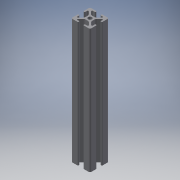
# Autodesk Inventor part: 25-2525_165mm
Saved by Autodesk Inventor 2019.4 (Build 234330000, 330)
## iProperties
Company: 80/20 Inc.
Created: 2014-04-23
Part Number: 25-2525_165mm
Material: Generic
Document SubType Name: Modeling
Designer: Ross Bowman
Density: 1 g/cm^3
Engineer: Ross Bowman
Catalog Web Link: 8020.net
Vendor: 80/20 Inc.
Appearance: Default
Material: 6105-T5 Aluminum
Author: Ross Bowman
Keywords: 80/20 , 8020 , T-Slot , Extrusion
Autodesk Inventor part; units mm, degrees
ref_plane "YZ Plane" through (0, 0, 0) normal (1, 0, 0) x (0, 1, 0)
ref_plane "XZ Plane" through (0, 0, 0) normal (0, 1, 0) x (-1, 0, 0)
ref_plane "XY Plane" through (0, 0, 0) normal (0, 0, 1) x (1, 0, 0)
sketch "Sketch1" plane through (0, 0, 0) normal (0, 0, 1) x (1, 0, 0)
  circle A0 centre (0, 0) radius 2.5
  arc A1 (-8.6363, 7.1116) -> (-10.36, 6.3969) centre (-9.35, 6.3969) ccw
  line L0 (-8.6363, 7.1116) -> (-5.4322, 3.9121)
  arc A2 (-4.455, 1.5554) -> (-5.4322, 3.9121) centre (-7.7855, 1.5554) ccw
  line L1 (-4.455, 1.5554) -> (-4.455, -1.5554)
  arc A3 (-5.4322, -3.9121) -> (-4.455, -1.5554) centre (-7.7855, -1.5554) ccw
  line L2 (-5.4322, -3.9121) -> (-8.6363, -7.1116)
  arc A4 (-10.36, -6.3969) -> (-8.6363, -7.1116) centre (-9.35, -6.3969) ccw
  line L3 (-10.36, -6.3969) -> (-10.36, -4.32)
  arc A5 (-10.36, -4.32) -> (-12.5, -4.32) centre (-11.43, -4.32) ccw
  line L4 (-12.5, -4.32) -> (-12.5, -10.5371)
  arc A6 (-12.5, -10.5371) -> (-10.5371, -12.5) centre (-10.5371, -10.5371) ccw
  line L5 (-10.5371, -12.5) -> (-4.3879, -12.5)
  arc A7 (-4.3879, -12.5) -> (-4.3879, -10.36) centre (-4.3879, -11.43) ccw
  line L6 (-4.3879, -10.36) -> (-6.42, -10.36)
  arc A8 (-7.1337, -8.6353) -> (-6.42, -10.36) centre (-6.42, -9.35) ccw
  line L7 (-7.1337, -8.6353) -> (-3.7953, -5.3018)
  arc A9 (-1.5554, -4.375) -> (-3.7953, -5.3018) centre (-1.5554, -7.545) ccw
  line L8 (-1.5554, -4.375) -> (1.5554, -4.375)
  arc A10 (3.7953, -5.3018) -> (1.5554, -4.375) centre (1.5554, -7.545) ccw
  line L9 (3.7953, -5.3018) -> (7.1337, -8.6353)
  arc A11 (6.42, -10.36) -> (7.1337, -8.6353) centre (6.42, -9.35) ccw
  line L10 (6.42, -10.36) -> (4.3879, -10.36)
  arc A12 (4.3879, -10.36) -> (4.3879, -12.5) centre (4.3879, -11.43) ccw
  line L11 (4.3879, -12.5) -> (10.5371, -12.5)
  arc A13 (10.5371, -12.5) -> (12.5, -10.5371) centre (10.5371, -10.5371) ccw
  line L12 (12.5, -10.5371) -> (12.5, -4.32)
  arc A14 (12.5, -4.32) -> (10.36, -4.32) centre (11.43, -4.32) ccw
  line L13 (10.36, -4.32) -> (10.36, -6.3969)
  arc A15 (8.6363, -7.1116) -> (10.36, -6.3969) centre (9.35, -6.3969) ccw
  line L14 (8.6363, -7.1116) -> (5.4322, -3.9121)
  arc A16 (4.455, -1.5554) -> (5.4322, -3.9121) centre (7.7855, -1.5554) ccw
  line L15 (4.455, -1.5554) -> (4.455, 1.5554)
  arc A17 (5.4322, 3.9121) -> (4.455, 1.5554) centre (7.7855, 1.5554) ccw
  line L16 (5.4322, 3.9121) -> (8.6363, 7.1116)
  arc A18 (10.36, 6.3969) -> (8.6363, 7.1116) centre (9.35, 6.3969) ccw
  line L17 (10.36, 6.3969) -> (10.36, 4.32)
  arc A19 (10.36, 4.32) -> (12.5, 4.32) centre (11.43, 4.32) ccw
  line L18 (12.5, 4.32) -> (12.5, 10.5371)
  arc A20 (12.5, 10.5371) -> (10.5371, 12.5) centre (10.5371, 10.5371) ccw
  line L19 (10.5371, 12.5) -> (4.32, 12.5)
  arc A21 (4.32, 12.5) -> (4.32, 10.36) centre (4.32, 11.43) ccw
  line L20 (4.32, 10.36) -> (6.42, 10.36)
  arc A22 (7.1337, 8.6353) -> (6.42, 10.36) centre (6.42, 9.35) ccw
  line L21 (7.1337, 8.6353) -> (3.7953, 5.3018)
  arc A23 (1.5554, 4.375) -> (3.7953, 5.3018) centre (1.5554, 7.545) ccw
  line L22 (1.5554, 4.375) -> (-1.5554, 4.375)
  arc A24 (-3.7953, 5.3018) -> (-1.5554, 4.375) centre (-1.5554, 7.545) ccw
  line L23 (-3.7953, 5.3018) -> (-7.1337, 8.6353)
  arc A25 (-6.42, 10.36) -> (-7.1337, 8.6353) centre (-6.42, 9.35) ccw
  line L24 (-6.42, 10.36) -> (-4.32, 10.36)
  arc A26 (-4.32, 10.36) -> (-4.32, 12.5) centre (-4.32, 11.43) ccw
  line L25 (-4.32, 12.5) -> (-10.5371, 12.5)
  arc A27 (-10.5371, 12.5) -> (-12.5, 10.5371) centre (-10.5371, 10.5371) ccw
  line L26 (-12.5, 10.5371) -> (-12.5, 4.32)
  arc A28 (-12.5, 4.32) -> (-10.36, 4.32) centre (-11.43, 4.32) ccw
  line L27 (-10.36, 4.32) -> (-10.36, 6.3969)
  constraints: 56 end point, 56 point on circle, 29 centre point
extrude "Extrusion1" add sketch "Sketch1" against normal blind 100
move faces "Move1" translate (0, 0, 50) faces at (-7.171, 11.7774, 0)
move faces "Move2" translate (0, 0, 15) faces at (-7.171, 11.7774, 50)
body "Solid1"
